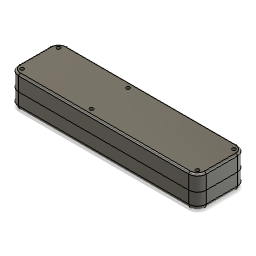
5ButtonKeyboard v4 (Autodesk Fusion 360 design; units mm, degrees)
Autodesk Fusion 360 part; units mm, degrees
sketch "Sketch Front" plane through (0, 0, 0) normal (0, 1, 0) x (1, 0, 0)
  circle A0 centre (0, 0) radius 9
  line L0 (-6, 3.6056) -> (-6, -3.6056)
  arc A1 (-6, -3.6056) -> (-6, 3.6056) centre (0, 0) ccw
  line L1 (-5.6, 2.1541) -> (-5.6, -2.1541)
  line L2 (5.6, 2.1541) -> (5.6, -2.1541)
  arc A2 (-5.6, -2.1541) -> (5.6, -2.1541) centre (0, 0) ccw
  arc A3 (5.6, 2.1541) -> (-5.6, 2.1541) centre (0, 0) ccw
  arc A4 (-45.6, -2.1541) -> (-34.4, -2.1541) centre (-40, 0) ccw
  circle A5 centre (-40, 0) radius 9
  line L3 (-46, 3.6056) -> (-46, -3.6056)
  arc A6 (-34.4, 2.1541) -> (-45.6, 2.1541) centre (-40, 0) ccw
  line L4 (-45.6, 2.1541) -> (-45.6, -2.1541)
  arc A7 (-46, -3.6056) -> (-46, 3.6056) centre (-40, 0) ccw
  line L5 (-34.4, 2.1541) -> (-34.4, -2.1541)
  arc A8 (-25.6, -2.1541) -> (-14.4, -2.1541) centre (-20, 0) ccw
  circle A9 centre (-20, 0) radius 9
  line L6 (-26, 3.6056) -> (-26, -3.6056)
  arc A10 (-14.4, 2.1541) -> (-25.6, 2.1541) centre (-20, 0) ccw
  line L7 (-25.6, 2.1541) -> (-25.6, -2.1541)
  arc A11 (-26, -3.6056) -> (-26, 3.6056) centre (-20, 0) ccw
  line L8 (-14.4, 2.1541) -> (-14.4, -2.1541)
  arc A12 (14.4, -2.1541) -> (25.6, -2.1541) centre (20, 0) ccw
  circle A13 centre (20, 0) radius 9
  line L9 (14, 3.6056) -> (14, -3.6056)
  arc A14 (25.6, 2.1541) -> (14.4, 2.1541) centre (20, 0) ccw
  line L10 (14.4, 2.1541) -> (14.4, -2.1541)
  arc A15 (14, -3.6056) -> (14, 3.6056) centre (20, 0) ccw
  line L11 (25.6, 2.1541) -> (25.6, -2.1541)
  arc A16 (34.4, -2.1541) -> (45.6, -2.1541) centre (40, 0) ccw
  circle A17 centre (40, 0) radius 9
  line L12 (34, 3.6056) -> (34, -3.6056)
  arc A18 (45.6, 2.1541) -> (34.4, 2.1541) centre (40, 0) ccw
  line L13 (34.4, 2.1541) -> (34.4, -2.1541)
  arc A19 (34, -3.6056) -> (34, 3.6056) centre (40, 0) ccw
  line L14 (45.6, 2.1541) -> (45.6, -2.1541)
  line L15 (-49, 14) -> (49, 14)
  line L16 (54, 9) -> (54, -9)
  line L17 (49, -14) -> (-49, -14)
  line L18 (-54, -9) -> (-54, 9)
  line L19 (-48.5, 12) -> (-13, 12)
  line L20 (52, 8.3) -> (52, -8)
  line L21 (-12.8, -12) -> (-48.5, -12)
  line L22 (-52, -10) -> (-52, 10)
  arc A20 (50, -12) -> (52, -10) centre (50, -10) ccw
  arc A21 (49, -14) -> (54, -9) centre (49, -9) ccw
  arc A22 (52, 10) -> (50, 12) centre (50, 10) ccw
  arc A23 (54, 9) -> (49, 14) centre (49, 9) ccw
  arc A24 (-50, 12) -> (-52, 10) centre (-50, 10) ccw
  arc A25 (-49, 14) -> (-54, 9) centre (-49, 9) ccw
  arc A26 (-52, -10) -> (-50, -12) centre (-50, -10) ccw
  arc A27 (-54, -9) -> (-49, -14) centre (-49, -9) ccw
  line L23 (-11.5, -9) -> (-9.5, -9)
  line L24 (-9, -9.5) -> (-9, -11)
  line L25 (-12, -11.2) -> (-12, -9.5)
  line L26 (-11.5, 9) -> (-9.5, 9)
  line L27 (-9, 9.5) -> (-9, 11)
  line L28 (-12, 11) -> (-12, 9.5)
  arc A28 (-12.8, -12) -> (-12, -11.2) centre (-12.8, -11.2) ccw
  line L29 (-8, -12) -> (48, -12)
  arc A29 (-9, -11) -> (-8, -12) centre (-8, -11) ccw
  arc A30 (-11.5, -9) -> (-12, -9.5) centre (-11.5, -9.5) ccw
  arc A31 (-9, -9.5) -> (-9.5, -9) centre (-9.5, -9.5) ccw
  arc A32 (-12, 11) -> (-13, 12) centre (-13, 11) ccw
  line L30 (48.3, 12) -> (-8, 12)
  arc A33 (-8, 12) -> (-9, 11) centre (-8, 11) ccw
  arc A34 (-12, 9.5) -> (-11.5, 9) centre (-11.5, 9.5) ccw
  arc A35 (-9.5, 9) -> (-9, 9.5) centre (-9.5, 9.5) ccw
  line L31 (-8, 12) -> (-13, 12)
  line L32 (-12.8, -12) -> (-8, -12)
  line L33 (-49.5, 9) -> (-52, 9)
  line L34 (-49, 11.5) -> (-49, 9.5)
  line L35 (-49.5, -9) -> (-52, -9)
  line L36 (-49, -11.5) -> (-49, -9.5)
  line L37 (49.5, -9) -> (51, -9)
  line L38 (49, -11) -> (49, -9.5)
  line L39 (49.6, 9) -> (51.3, 9)
  line L40 (49, 11.3) -> (49, 9.6)
  arc A36 (48, -12) -> (49, -11) centre (48, -11) ccw
  arc A37 (51, -9) -> (52, -8) centre (51, -8) ccw
  line L41 (52, -10) -> (52, -7.5)
  line L42 (48, -12) -> (50, -12)
  arc A38 (49.5, -9) -> (49, -9.5) centre (49.5, -9.5) ccw
  arc A39 (52, 8.3) -> (51.3, 9) centre (51.3, 8.3) ccw
  arc A40 (49, 11.3) -> (48.3, 12) centre (48.3, 11.3) ccw
  line L43 (52, 8.3) -> (52, 10)
  line L44 (48.3, 12) -> (50, 12)
  arc A41 (49, 9.6) -> (49.6, 9) centre (49.6, 9.6) ccw
  arc A42 (-48.5, 12) -> (-49, 11.5) centre (-48.5, 11.5) ccw
  arc A43 (-49.5, 9) -> (-49, 9.5) centre (-49.5, 9.5) ccw
  line L45 (-48.5, 12) -> (-50, 12)
  arc A44 (-49, -11.5) -> (-48.5, -12) centre (-48.5, -11.5) ccw
  line L46 (-48.5, -12) -> (-50, -12)
  arc A45 (-49, -9.5) -> (-49.5, -9) centre (-49.5, -9.5) ccw
  line L47 (-54, 4) -> (-52, 4)
  line L48 (-52, 4) -> (-52, -4)
  line L49 (-52, -4) -> (-54, -4)
  line L50 (-54, -4) -> (-54, 4)
  line L51 (-52, 4) -> (-50, 4)
  line L52 (-50, 4) -> (-50, 6)
  line L53 (-50, 6) -> (-52, 6)
  line L54 (-52, 6) -> (-52, 4)
  line L55 (-52, -4) -> (-50, -4)
  line L56 (-50, -4) -> (-50, -6)
  line L57 (-50, -6) -> (-52, -6)
  line L58 (-52, -6) -> (-52, -4)
  circle A46 centre (-10.5, -10.5) radius 0.65
  circle A47 centre (-50.5, -10.5) radius 0.65
  circle A48 centre (-50.5, 10.5) radius 0.65
  circle A49 centre (-10.5, 10.5) radius 0.65
  circle A50 centre (50.5, 10.5) radius 0.65
  circle A51 centre (50.5, -10.5) radius 0.65
  point P0 (-40, 0)
  point P1 (-20, 0)
  point P2 (20, 0)
  point P3 (40, 0)
  point P4 (-54, 14)
  point P5 (54, 14)
  point P6 (-54, -14)
  point P7 (-52, 12)
  point P8 (52, 12)
  point P9 (-52, -12)
  point P10 (-12, -9)
  point P11 (-9, -9)
  point P12 (-12, 9)
  point P13 (-9, 9)
  point P14 (52, 4)
  point P15 (52, -4)
  dimension "d1" = 18
  dimension "d2" = 14
  dimension "d3" = 6
  dimension "d4" = 12
  dimension "d5" = 5.6
  dimension "d6" = 5.6
  dimension "d9" = 20
  dimension "d10" = 0
  dimension "d13" = 108
  dimension "d14" = 28
  dimension "d15" = 54
  dimension "d16" = 14
  dimension "d17" = 104
  dimension "d18" = 24
  dimension "d19" = 2
  dimension "d20" = 2
  dimension "d107" = 2
  dimension "d108" = 5
  dimension "d109" = 2
  dimension "d110" = 5
  dimension "d111" = 2
  dimension "d112" = 5
  dimension "d113" = 2
  dimension "d114" = 5
  dimension "d118" = 3
  dimension "d119" = 3
  dimension "d121" = 1
  dimension "d122" = 0.5
  dimension "d123" = 0.5
  dimension "d124" = 1
  dimension "d125" = 1
  dimension "d126" = 0.5
  dimension "d127" = 1
  dimension "d128" = 0.5
  dimension "d129" = 0.7
  dimension "d130" = 0.7
  dimension "d131" = 0.6
  dimension "d132" = 0.5
  dimension "d133" = 0.5
  dimension "d134" = 0.5
  dimension "d135" = 8
  dimension "d136" = 10
  dimension "d137" = 1.3
  dimension "d138" = 1.3
  dimension "d139" = 1.3
  dimension "d140" = 1.3
  dimension "d141" = 1.3
  dimension "d142" = 1.3
  constraint coincident A0.centre A1.centre
  constraint concentric A0 A1
  constraint vertical L0
  constraint vertical L1
  constraint coincident L2.start A2
  constraint vertical L2
  constraint concentric A2 A3
  constraint horizontal L15
  constraint vertical L16
  constraint horizontal L17
  constraint vertical L18
  constraint horizontal L19
  constraint vertical L20
  constraint horizontal L21
  constraint vertical L22
  constraint tangent L20 A20
  constraint tangent L21 A20
  constraint tangent L16 A21
  constraint tangent L17 A21
  constraint coincident P8 L19
  constraint coincident P8 L20
  constraint tangent L19 A22
  constraint tangent L20 A22
  constraint coincident P5 L15
  constraint coincident P5 L16
  constraint tangent L15 A23
  constraint tangent L16 A23
  constraint coincident P7 L19
  constraint coincident P7 L22
  constraint tangent L19 A24
  constraint tangent L22 A24
  constraint coincident P4 L15
  constraint coincident P4 L18
  constraint tangent L15 A25
  constraint tangent L18 A25
  constraint coincident P9 L21
  constraint coincident P9 L22
  constraint tangent L21 A26
  constraint tangent L22 A26
  constraint coincident P6 L17
  constraint coincident P6 L18
  constraint tangent L17 A27
  constraint tangent L18 A27
  constraint horizontal L23
  constraint vertical L24
  constraint vertical L25
  constraint horizontal L26
  constraint vertical L27
  constraint vertical L28
  constraint coincident L21 A20.start
  constraint tangent L21 A28
  constraint tangent L25 A28
  constraint tangent L24 A29
  constraint tangent L29 A29
  constraint coincident P10 L23
  constraint coincident P10 L25
  constraint tangent L23 A30
  constraint tangent L25 A30
  constraint coincident P11 L23
  constraint coincident P11 L24
  constraint tangent L23 A31
  constraint tangent L24 A31
  constraint coincident L19 A22.end
  constraint tangent L19 A32
  constraint tangent L28 A32
  constraint tangent A22 L30
  constraint tangent L27 A33
  constraint tangent L30 A33
  constraint coincident P12 L26
  constraint coincident P12 L28
  constraint tangent L26 A34
  constraint tangent L28 A34
  constraint coincident P13 L26
  constraint coincident P13 L27
  constraint tangent L26 A35
  constraint tangent L27 A35
  constraint equal A34 A35
  constraint tangent A29 L32
  constraint horizontal L33
  constraint vertical L34
  constraint horizontal L35
  constraint vertical L36
  constraint horizontal L37
  constraint vertical L38
  constraint horizontal L39
  constraint vertical L40
  constraint coincident A20.start L29
  constraint tangent L29 A36
  constraint tangent L38 A36
  constraint coincident L20 A20.end
  constraint tangent L20 A37
  constraint tangent L37 A37
  constraint equal A36 A37
  constraint coincident L20 L41.end
  constraint parallel L20 L41
  constraint tangent A20 L42
  constraint tangent L37 A38
  constraint tangent L38 A38
  constraint coincident L20 A22.start
  constraint tangent L20 A39
  constraint tangent L39 A39
  constraint coincident A22.end L30
  constraint tangent L30 A40
  constraint tangent L40 A40
  constraint tangent L39 A41
  constraint tangent L40 A41
  constraint coincident L19 A24.start
  constraint tangent L34 A42
  constraint tangent L19 A42
  constraint tangent L33 A43
  constraint tangent L34 A43
  constraint equal A42 A43
  constraint coincident L21 A26.end
  constraint tangent L21 A44
  constraint tangent L36 A44
  constraint tangent L35 A45
  constraint tangent L36 A45
  constraint horizontal L47
  constraint vertical L48
  constraint horizontal L49
  constraint vertical L50
  constraint coincident L18 L47.start
  constraint horizontal L51
  constraint vertical L52
  constraint horizontal L53
  constraint vertical L54
  constraint horizontal L55
  constraint vertical L56
  constraint horizontal L57
  constraint vertical L58
  measures "d1" diameter of A0
  measures "d2" diameter of A1
  measures "d3" distance of A0.centre L0
  measures "d4" diameter of A2
  measures "d5" distance of A0.centre L1
  measures "d6" distance of A0.centre L2
  measures "d13" distance of P4 P5
  measures "d14" distance of P4 P6
  measures "d15" distance of A0.centre L18
  measures "d16" distance of P0 L15
  measures "d17" distance of P7 P8
  measures "d18" distance of P7 P9
  measures "d19" distance of L15 L19
  measures "d20" distance of L18 L22
  measures "d107" radius of A20
  measures "d108" radius of A21
  measures "d109" radius of A22
  measures "d110" radius of A23
  measures "d111" radius of A24
  measures "d112" radius of A25
  measures "d113" radius of A26
  measures "d114" radius of A27
  measures "d118" distance of P10 P11
  measures "d119" distance of P12 P13
  measures "d121" radius of A29
  measures "d122" radius of A30
  measures "d123" radius of A31
  measures "d124" radius of A32
  measures "d125" radius of A33
  measures "d126" radius of A34
  measures "d127" radius of A36
  measures "d128" radius of A38
  measures "d129" radius of A39
  measures "d130" radius of A40
  measures "d131" radius of A41
  measures "d132" radius of A42
  measures "d133" radius of A44
  measures "d134" radius of A45
  measures "d135" distance of L47.start L49.end
  measures "d136" distance of L15 L47
  measures "d137" diameter of A46
  measures "d138" diameter of A47
  measures "d139" diameter of A48
  measures "d140" diameter of A49
  measures "d141" diameter of A50
  measures "d142" diameter of A51
sketch "Sketch Back" plane through (0, 17, 0) normal (0, 1, 0) x (-1, 0, 0)
  line L0 (49, 14) -> (-49, 14)
  line L1 (-54, 9) -> (-54, -9)
  line L2 (-49, -14) -> (49, -14)
  line L3 (19, 9) -> (52, 9) construction
  line L4 (19, -9) -> (19, 9) construction
  line L5 (52, -9) -> (19, -9) construction
  line L6 (52, 9) -> (52, -9) construction
  line L7 (19, 9) -> (16, 9)
  line L8 (16, 9) -> (16, -9)
  line L9 (16, -9) -> (19, -9)
  line L10 (19, -9) -> (19, 9)
  line L11 (54, 4) -> (52, 4)
  line L12 (52, 4) -> (52, -4)
  line L13 (52, -4) -> (54, -4)
  line L14 (54, -4) -> (54, 4)
  line L15 (13, 11.2) -> (48.3, 11.2)
  line L16 (48.5, -11.2) -> (13, -11.2)
  line L17 (-51.2, -8.3) -> (-51.2, 8)
  line L18 (51.2, 9) -> (52, 9)
  line L19 (51.2, -9) -> (52, -9)
  line L20 (50, -12) -> (49, -12)
  line L21 (49, -10.7) -> (49, -9.4)
  line L22 (49.4, -9) -> (52, -9)
  line L23 (52, -9) -> (52, -10)
  line L24 (50, 12) -> (49, 12)
  line L25 (49, 10.5) -> (49, 9)
  line L26 (49, 9) -> (52, 9)
  line L27 (52, 9) -> (52, 10)
  line L28 (-50, -12) -> (-49, -12)
  line L29 (-49, -10.5) -> (-49, -9.4)
  line L30 (-49.4, -9) -> (-50.5, -9)
  line L31 (-52, -9) -> (-52, -10)
  line L32 (-50, 12) -> (-49, 12)
  line L33 (-49, 10.2) -> (-49, 9.3)
  line L34 (-49.3, 9) -> (-50.2, 9)
  line L35 (-52, 9) -> (-52, 10)
  arc A0 (-48, 11.2) -> (-49, 10.2) centre (-48, 10.2) ccw
  arc A1 (-50.2, 9) -> (-51.2, 8) centre (-50.2, 8) ccw
  arc A2 (-50, 12) -> (-52, 10) centre (-50, 10) ccw
  arc A3 (-49.3, 9) -> (-49, 9.3) centre (-49.3, 9.3) ccw
  line L36 (51.2, 9) -> (49, 9)
  arc A4 (49, 10.5) -> (48.3, 11.2) centre (48.3, 10.5) ccw
  arc A5 (-51.2, -8.3) -> (-50.5, -9) centre (-50.5, -8.3) ccw
  arc A6 (-49, -10.5) -> (-48.3, -11.2) centre (-48.3, -10.5) ccw
  arc A7 (-52, -10) -> (-50, -12) centre (-50, -10) ccw
  arc A8 (-49, -9.4) -> (-49.4, -9) centre (-49.4, -9.4) ccw
  line L37 (49, -14) -> (-49, -14)
  line L38 (-54, -9) -> (-54, 9)
  line L39 (-49, 14) -> (49, 14)
  arc A9 (-54, -9) -> (-49, -14) centre (-49, -9) ccw
  arc A10 (-49, 14) -> (-54, 9) centre (-49, 9) ccw
  arc A11 (48.5, -11.2) -> (49, -10.7) centre (48.5, -10.7) ccw
  arc A12 (50, -12) -> (52, -10) centre (50, -10) ccw
  arc A13 (49, -14) -> (54, -9) centre (49, -9) ccw
  arc A14 (49.4, -9) -> (49, -9.4) centre (49.4, -9.4) ccw
  arc A15 (52, 10) -> (50, 12) centre (50, 10) ccw
  arc A16 (54, 9) -> (49, 14) centre (49, 9) ccw
  line L40 (-49, -12) -> (49, -12)
  line L41 (49, 12) -> (-49, 12)
  line L42 (-52, 9) -> (-52, -9)
  line L43 (54, 9) -> (54, -9)
  arc A17 (-49, 14) -> (-54, 9) centre (-49, 9) ccw
  arc A18 (-54, -9) -> (-49, -14) centre (-49, -9) ccw
  arc A19 (49, -14) -> (54, -9) centre (49, -9) ccw
  arc A20 (54, 9) -> (49, 14) centre (49, 9) ccw
  line L44 (11.7, -9) -> (9.3, -9)
  line L45 (9, -9.3) -> (9, -10.2)
  line L46 (9, -12) -> (12, -12)
  line L47 (12, -10.2) -> (12, -9.3)
  line L48 (11.7, 9) -> (9.3, 9)
  line L49 (9, 9.3) -> (9, 10.2)
  line L50 (9, 12) -> (12, 12)
  line L51 (12, 10.2) -> (12, 9.3)
  circle A21 centre (10.5, 10.5) radius 0.7
  circle A22 centre (10.5, 10.5) radius 1
  circle A23 centre (50.5, 10.5) radius 0.7
  circle A24 centre (50.5, 10.5) radius 1
  circle A25 centre (50.5, -10.5) radius 0.7
  circle A26 centre (50.5, -10.5) radius 1
  circle A27 centre (10.5, -10.5) radius 0.7
  circle A28 centre (10.5, -10.5) radius 1
  circle A29 centre (-50.5, 10.5) radius 0.7
  circle A30 centre (-50.5, 10.5) radius 1
  circle A31 centre (-50.5, -10.5) radius 0.7
  circle A32 centre (-50.5, -10.5) radius 1
  arc A33 (12, -10.2) -> (13, -11.2) centre (13, -10.2) ccw
  line L52 (-48.3, -11.2) -> (8, -11.2)
  arc A34 (8, -11.2) -> (9, -10.2) centre (8, -10.2) ccw
  arc A35 (12, -9.3) -> (11.7, -9) centre (11.7, -9.3) ccw
  arc A36 (9.3, -9) -> (9, -9.3) centre (9.3, -9.3) ccw
  arc A37 (13, 11.2) -> (12, 10.2) centre (13, 10.2) ccw
  line L53 (-48, 11.2) -> (8, 11.2)
  arc A38 (9, 10.2) -> (8, 11.2) centre (8, 10.2) ccw
  arc A39 (11.7, 9) -> (12, 9.3) centre (11.7, 9.3) ccw
  arc A40 (9, 9.3) -> (9.3, 9) centre (9.3, 9.3) ccw
  line L54 (52, 9) -> (52, 4)
  line L55 (52, -4) -> (52, -9)
  point P0 (52, -12)
  point P1 (52, 12)
  point P2 (-52, -12)
  point P3 (-52, 12)
  point P4 (12, -9)
  point P5 (9, -9)
  point P6 (12, 9)
  point P7 (9, 9)
  dimension "d27" = 33
  dimension "d28" = 18
  dimension "d35" = 3
  dimension "d36" = 18
  dimension "d69" = 2
  dimension "d70" = 8
  dimension "d85" = 3
  dimension "d86" = 3
  dimension "d87" = 3
  dimension "d88" = 3
  dimension "d89" = 3
  dimension "d90" = 3
  dimension "d91" = 1
  dimension "d93" = 2
  dimension "d94" = 0.3
  dimension "d95" = 0.7
  dimension "d97" = 2
  dimension "d98" = 0.4
  dimension "d99" = 5
  dimension "d100" = 5
  dimension "d101" = 0.5
  dimension "d102" = 2
  dimension "d103" = 5
  dimension "d104" = 0.4
  dimension "d105" = 2
  dimension "d106" = 5
  dimension "d115" = 3
  dimension "d116" = 3
  dimension "d117" = 3
  dimension "d143" = 1.4
  dimension "d144" = 2
  dimension "d145" = 1.4
  dimension "d146" = 2
  dimension "d147" = 1.4
  dimension "d148" = 2
  dimension "d149" = 1.4
  dimension "d150" = 2
  dimension "d151" = 1.4
  dimension "d152" = 2
  dimension "d153" = 1.4
  dimension "d154" = 2
  dimension "d157" = 1
  dimension "d158" = 1
  dimension "d159" = 0.3
  dimension "d160" = 0.3
  dimension "d161" = 1
  dimension "d162" = 1
  dimension "d163" = 0.3
  constraint horizontal L3
  constraint vertical L6
  constraint horizontal L5
  constraint vertical L4
  constraint horizontal L7
  constraint vertical L8
  constraint horizontal L9
  constraint vertical L10
  constraint horizontal L11
  constraint vertical L12
  constraint horizontal L13
  constraint vertical L14
  constraint coincident L3 L18.start
  constraint coincident L5 L19.start
  constraint horizontal L20
  constraint vertical L21
  constraint horizontal L22
  constraint vertical L23
  constraint horizontal L24
  constraint vertical L25
  constraint horizontal L26
  constraint vertical L27
  constraint horizontal L28
  constraint vertical L29
  constraint horizontal L30
  constraint vertical L31
  constraint horizontal L32
  constraint vertical L33
  constraint horizontal L34
  constraint vertical L35
  constraint coincident L32.end L33
  constraint tangent L15 A0
  constraint tangent L33 A0
  constraint coincident L35.start L34
  constraint tangent L34 A1
  constraint tangent L17 A1
  constraint equal A0 A1
  constraint coincident P3 L32
  constraint coincident P3 L35
  constraint tangent L32 A2
  constraint tangent L35 A2
  constraint tangent L34 A3
  constraint tangent L33 A3
  constraint perpendicular L25 L36
  constraint coincident L24.end L25
  constraint tangent L15 A4
  constraint tangent L25 A4
  constraint coincident L31.start L30
  constraint tangent L17 A5
  constraint tangent L30 A5
  constraint equal A4 A5
  constraint coincident L28.end L29
  constraint tangent L29 A6
  constraint tangent L16 A6
  constraint equal A4 A6
  constraint coincident P2 L31
  constraint coincident P2 L28
  constraint tangent L31 A7
  constraint tangent L28 A7
  constraint tangent L30 A8
  constraint tangent L29 A8
  constraint tangent L38 A9
  constraint tangent L37 A9
  constraint tangent L39 A10
  constraint tangent L38 A10
  constraint coincident L20.end L21
  constraint tangent L21 A11
  constraint tangent L16 A11
  constraint coincident P0 L23
  constraint coincident P0 L20
  constraint tangent L23 A12
  constraint tangent L20 A12
  constraint tangent L37 A13
  constraint tangent L21 A14
  constraint tangent L22 A14
  constraint coincident P1 L24
  constraint coincident P1 L27
  constraint tangent L24 A15
  constraint tangent L27 A15
  constraint tangent L39 A16
  constraint tangent A13 L43
  constraint horizontal L44
  constraint vertical L45
  constraint horizontal L46
  constraint vertical L47
  constraint horizontal L48
  constraint vertical L49
  constraint horizontal L50
  constraint vertical L51
  constraint coincident L41 L50.start
  constraint concentric A21 A22
  constraint concentric A23 A24
  constraint concentric A25 A26
  constraint concentric A27 A28
  constraint concentric A29 A30
  constraint concentric A31 A32
  constraint coincident L16 A6.end
  constraint coincident L46.end L47
  constraint tangent L16 A33
  constraint tangent L47 A33
  constraint tangent A6 L52
  constraint perpendicular L45 L52
  constraint coincident L46.start L45
  constraint tangent L52 A34
  constraint tangent L45 A34
  constraint coincident P4 L44
  constraint coincident P4 L47
  constraint tangent L44 A35
  constraint tangent L47 A35
  constraint coincident P5 L44
  constraint coincident P5 L45
  constraint tangent L44 A36
  constraint tangent L45 A36
  constraint coincident L15 A0.start
  constraint coincident L50.end L51
  constraint tangent L15 A37
  constraint tangent L51 A37
  constraint tangent A0 L53
  constraint perpendicular L49 L53
  constraint coincident L50.start L49
  constraint tangent L49 A38
  constraint tangent L53 A38
  constraint coincident P6 L48
  constraint coincident P6 L51
  constraint tangent L48 A39
  constraint tangent L51 A39
  constraint coincident P7 L48
  constraint coincident P7 L49
  constraint tangent L48 A40
  constraint tangent L49 A40
  constraint equal A39 A40
  constraint perpendicular L3 L54
  measures "d27" distance of L3.start L3.end
  measures "d28" distance of L3.start L4.start
  measures "d35" distance of L3.start L7.end
  measures "d36" distance of L3.start L4.start
  measures "d69" distance of L11.start L11.end
  measures "d70" distance of L11.start L13.end
  measures "d85" distance of P0 L20.end
  measures "d86" distance of P1 L24.end
  measures "d87" distance of P2 L28.end
  measures "d88" distance of P2 L31.start
  measures "d89" distance of P3 L32.end
  measures "d90" distance of P3 L35.start
  measures "d91" radius of A0
  measures "d93" radius of A2
  measures "d94" radius of A3
  measures "d95" radius of A4
  measures "d97" radius of A7
  measures "d98" radius of A8
  measures "d99" radius of A9
  measures "d100" radius of A10
  measures "d101" radius of A11
  measures "d102" radius of A12
  measures "d103" radius of A13
  measures "d104" radius of A14
  measures "d105" radius of A15
  measures "d106" radius of A16
  measures "d115" distance of P4 P5
  measures "d116" distance of P4 L46.end
  measures "d117" distance of P6 P7
  measures "d143" diameter of A21
  measures "d144" diameter of A22
  measures "d145" diameter of A23
  measures "d146" diameter of A24
  measures "d147" diameter of A25
  measures "d148" diameter of A26
  measures "d149" diameter of A27
  measures "d150" diameter of A28
  measures "d151" diameter of A29
  measures "d152" diameter of A30
  measures "d153" diameter of A31
  measures "d154" diameter of A32
  measures "d157" radius of A33
  measures "d158" radius of A34
  measures "d159" radius of A35
  measures "d160" radius of A36
  measures "d161" radius of A37
  measures "d162" radius of A38
  measures "d163" radius of A39
extrude "Extrude12" add sketch "Sketch Front" along normal blind 2 contours L15 L16 L17 L18 L19 L20 L21 L22 A20 A21 A22 A23 A24 A25 A26 A27 L29 L30 L31 L32 L41 L42 L43 L44 L45 L46 L47 L49 L54 L58 | L18 L22 L47 L48 L49 L50 | L19 L20 L21 L22 L23 L24 L25 L26 L27 L28 A28 L29 A29 A30 A31 A32 L30 A33 A34 A35 L33 L34 L35 L36 L37 L38 L39 L40 A36 A37 L41 A38 A39 A40 A41 A42 A43 A44 A45 L48 L51 L52 L53 L55 L56 L57 | L22 L51 L52 L53 L54 | L22 L55 L56 L57 L58 | L22 A24 L33 L34 A42 A43 L45 | L22 A26 L35 L36 A44 L46 A45 | L26 L27 L28 A32 A33 A34 A35 L31 | L23 L24 L25 A28 A29 A30 A31 L32 | A22 L39 L40 A39 A40 L43 L44 A41 | A20 L37 L38 A36 A37 L41 L42 A38 | A46 | A47 | A48 | A49 | A50 | A51 makes body 1
extrude "Extrude13" add sketch "Sketch Back" along normal blind 2 separate body contours L0 L1 L2 L11 L13 L20 L23 L24 L27 L28 L31 L32 L35 A2 A7 L37 L38 L39 A9 A10 A12 A13 A15 A16 L40 L41 L42 L43 A17 A18 A19 A20 L46 L50 L54 L55 | L11 L12 L13 L14 L43 | L12 L15 L16 L17 L18 L19 L21 L22 L25 L26 L29 L30 L33 L34 A0 A1 A3 L36 A4 A5 A6 A8 A11 A14 L44 L45 L47 L48 L49 L51 A33 L52 A34 A35 A36 A37 L53 A38 A39 A40 L54 L55 | L15 L16 L17 L18 L19 L20 L21 L22 L23 L24 L25 L26 L27 L28 L29 L30 L31 L32 L33 L34 L35 A0 A1 A2 A3 L36 A4 A5 A6 A7 A8 A11 A12 A14 A15 L40 L41 L42 L44 L45 L46 L47 L48 L49 L50 L51 A33 L52 A34 A35 A36 A37 L53 A38 A39 A40 | L7 L8 L9 L10 makes body 2
extrude "Extrude14" add sketch "Sketch Front" along normal blind 1.5 contours A0 | L0 A1 | A5 | L3 A7 | A9 | L6 A11 | A13 | L9 A15 | A17 | L12 A19 bodies 1
extrude "Extrude15" cut sketch "Sketch Front" along normal blind 0.2 contours L0 A1 | L3 A7 | L6 A11 | L9 A15 | L12 A19 bodies 1
extrude "Extrude16" add sketch "Sketch Front" along normal blind 10 contours L15 L16 L17 L18 L19 L20 L21 L22 A20 A21 A22 A23 A24 A25 A26 A27 L29 L30 L31 L32 L41 L42 L43 L44 L45 L46 L47 L49 L54 L58 bodies 1
extrude "Extrude17" add sketch "Sketch Back" against normal blind 7 contours L0 L1 L2 L11 L13 L20 L23 L24 L27 L28 L31 L32 L35 A2 A7 L37 L38 L39 A9 A10 A12 A13 A15 A16 L40 L41 L42 L43 A17 A18 A19 A20 L46 L50 L54 L55 bodies 2
extrude "Extrude18" add sketch "Sketch Back" against normal blind 9 contours L15 L16 L17 L18 L19 L20 L21 L22 L23 L24 L25 L26 L27 L28 L29 L30 L31 L32 L33 L34 L35 A0 A1 A2 A3 L36 A4 A5 A6 A7 A8 A11 A12 A14 A15 L40 L41 L42 L44 L45 L46 L47 L48 L49 L50 L51 A33 L52 A34 A35 A36 A37 L53 A38 A39 A40 | A22 | A24 | A26 | A28 | A30 | A32 bodies 2
extrude "Extrude19" add sketch "Sketch Back" against normal blind 2 contours L11 L12 L13 L14 L43 bodies 2
extrude "Extrude20" add sketch "Sketch Back" against normal blind 4 contours L7 L8 L9 L10 bodies 2
chamfer "Chamfer3" distance 0.5 distance2 2 1 edges at (-19, 13, 0) measured on face at (-17, 13, 3) on bodies 2
extrude "Extrude21" add 1 faces at (-18.6667, 13.6667, 3) along direction (-0.970143, -0.242536, 0) blind 2 on bodies 2 bodies 2
fillet "Fillet10" radius 1 2 edges at (-20.9403, 14.5149, 0) (-20.4403, 12.5149, 0) on bodies 2
fillet "Fillet11" radius 1 8 edges at (0, 19, 14) (52.5355, 19, 12.5355) (54, 19, 0) (52.5355, 19, -12.5355) (0, 19, -14) (-52.5355, 19, -12.5355) (-54, 19, 0) (-52.5355, 19, 12.5355) on bodies 2
extrude "Extrude22" add sketch "Sketch Front" along normal blind 8 contours L22 A24 L33 L34 A42 A43 L45 | L22 A26 L35 L36 A44 L46 A45 | L26 L27 L28 A32 A33 A34 A35 L31 | L23 L24 L25 A28 A29 A30 A31 L32 | A22 L39 L40 A39 A40 L43 L44 A41 | A20 L37 L38 A36 A37 L41 L42 A38 bodies 1
extrude "Extrude23" add sketch "Sketch Front" along normal blind 13 contours L18 L22 L47 L48 L49 L50 bodies 1
extrude "Extrude24" add sketch "Sketch Front" along normal blind 15 contours L22 L51 L52 L53 L54 | L22 L55 L56 L57 L58 bodies 1
fillet "Fillet12" radius 2 37 edges at (-50.75, 2, 9) (-49.1464, 2, 9.1464) (-49, 2, 10.5) (-48.8536, 2, 11.8536) (-30.65, 2, 12) (-12.2343, 2, 11.7657) (-12, 2, 10.35) (-11.8536, 2, 9.1464) (-10.5, 2, 9) (-9.1464, 2, 9.1464) (-9, 2, 10.25) (-8.7071, 2, 11.7071) (20, 2, 12) (48.7071, 2, 11.7071) (49, 2, 10.25) (49.1464, 2, 9.1464) (50.25, 2, 9) (51.7071, 2, 8.7071) (52, 2, -0.15) (51.795, 2, -8.795) (50.45, 2, -9) (49.1757, 2, -9.1757) (49, 2, -10.45) (48.795, 2, -11.795) (20.15, 2, -12) (-8.7071, 2, -11.7071) (-9, 2, -10.25) (-9.1464, 2, -9.1464) (-10.5, 2, -9) (-11.8536, 2, -9.1464) (-12, 2, -10.25) (-12.2929, 2, -11.7071) (-30.75, 2, -12) (-48.8536, 2, -11.8536) (-49, 2, -10.5) (-49.1464, 2, -9.1464) (-50.75, 2, -9) on bodies 1
fillet "Fillet13" radius 2 7 edges at (-52, 2, 0) (-52, 6, -9) (-52, 2.5858, -8.4142) (-52, 2, -6.5) (-52, 2, 6.5) (-52, 2.5858, 8.4142) (-52, 6, 9) on bodies 1
fillet "Fillet14" radius 1 4 edges at (-50, 15, -5) (-50, 15, 5) (-52, 15, 5) (-52, 15, -5) on bodies 1
fillet "Fillet15" radius 3 8 edges at (52.5355, 0, 12.5355) (0, 0, 14) (-52.5355, 0, 12.5355) (-54, 0, 0) (-52.5355, 0, -12.5355) (0, 0, -14) (52.5355, 0, -12.5355) (54, 0, 0) on bodies 1
extrude "Extrude25" cut 6 faces at (-11.3937, 17, 10.4155) (-50.2188, 17, 9.6475) (-49.6582, 17, -10.8117) (-11.3937, 17, -10.5845) (51.2126, 17, -9.9541) (51.2126, 17, 9.9541) along direction (0, -1, 0) blind 7.5 on bodies 2 bodies 2
equation "d6 = d5"
equation "d15 = d13 / 2"
equation "d16 = d14 / 2"
equation "d136 = ( d14 - d135 ) / 2"
named bodies: "Top", "Bottom"
